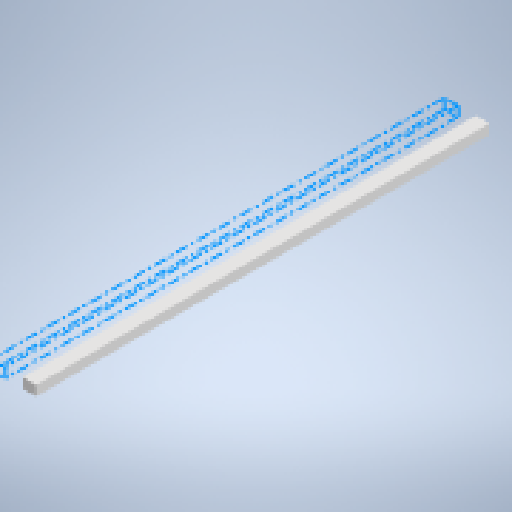
# Autodesk Inventor part: Rail
Saved by Autodesk Inventor 2023 (Build 270158000, 158)
## iProperties
Created: 2022-09-16
Part Number: Rail
Material: Generic
Document SubType Name: Modeling
Designer: deli
Density: 1 g/cm^3
Appearance: Default
Author: deli
Autodesk Inventor part; units mm, degrees
ref_plane "YZ Plane" through (0, 0, 0) normal (1, 0, 0) x (0, 1, 0)
ref_plane "XZ Plane" through (0, 0, 0) normal (0, 1, 0) x (-1, 0, 0)
ref_plane "XY Plane" through (0, 0, 0) normal (0, 0, 1) x (1, 0, 0)
sketch "Sketch4" plane through (0, 0, 0) normal (0, 0, 1) x (1, 0, 0)
  line L0 (-22.685, 6.9816) -> (-13.685, 6.9816)
  line L1 (-13.685, 6.9816) -> (-13.685, 0.4816)
  line L2 (-13.685, 0.4816) -> (-22.685, 0.4816)
  line L3 (-22.685, 0.4816) -> (-22.685, 6.9816)
  point P0 (0, 0)
  dimension "d27" = 9
  dimension "d28" = 6.5
  constraints: 8 end point, 2 parallel, 1 horizontal, 1 perpendicular
  measures "d27" distance of L1.end L2.end
  measures "d28" distance of L0.end L1.end
extrude "Extrusion3" add sketch "Sketch4" along normal blind 300
body "Solid2"
